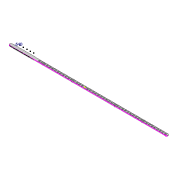
# Autodesk Inventor part: secondbow
Saved by Autodesk Inventor 2017 (Build 210142000, 142)
## iProperties
Created: 2017-04-15
Part Number: secondbow
Material: Generic
Document SubType Name: Modeling
Designer: Gideon
Density: 1 g/cm^3
Appearance: Default
Author: Gideon
Autodesk Inventor part; units mm, degrees
ref_plane "YZ Plane" through (0, 0, 0) normal (1, 0, 0) x (0, 1, 0)
ref_plane "XZ Plane" through (0, 0, 0) normal (0, 1, 0) x (-1, 0, 0)
ref_plane "XY Plane" through (0, 0, 0) normal (0, 0, 1) x (1, 0, 0)
sketch "Sketch1" plane through (0, 0, 0) normal (0, 0, 1) x (1, 0, 0)
  line L0 (-354.9792, 6.35) -> (394.3208, 6.35)
  line L1 (394.3208, 6.35) -> (394.3208, -6.35)
  line L2 (394.3208, -6.35) -> (-354.9792, -6.35)
  line L3 (-354.9792, -6.35) -> (-354.9792, 6.35)
  line L4 (-410.3367, 0) -> (469.0371, 0)
  point P0 (0, 0)
  dimension "d0" = 749.3
  dimension "d1" = 12.7
  constraints: 10 end point, 2 horizontal, 2 parallel, 1 perpendicular, 1 other
  measures "d0" distance of L0.end L0.start
  measures "d1" distance of L2.end L0.start
extrude "Extrusion1" add sketch "Sketch1" along normal blind 7.62
sketch "Sketch2" plane through (0, 0, 7.62) normal (0, 0, 1) x (1, 0, 0)
  line L0 (379.0808, 3.8322) -> (386.7008, 3.8322)
  line L1 (386.7008, 3.8322) -> (386.7008, -3.7878)
  line L2 (386.7008, -3.7878) -> (379.0808, -3.7878)
  line L3 (379.0808, -3.7878) -> (379.0808, 3.8322)
  line L4 (394.3208, -6.35) -> (394.3208, 6.35) projected
  line L5 (359.1521, 0.0222) -> (400.4054, 0.0222)
  line L6 (366.3808, -3.7878) -> (366.3808, 3.8322)
  line L7 (366.3808, 3.8322) -> (374.0008, 3.8322)
  line L8 (374.0008, 3.8322) -> (374.0008, -3.7878)
  line L9 (374.0008, -3.7878) -> (366.3808, -3.7878)
  line L10 (353.6808, -3.7878) -> (353.6808, 3.8322)
  line L11 (353.6808, 3.8322) -> (361.3008, 3.8322)
  line L12 (361.3008, 3.8322) -> (361.3008, -3.7878)
  line L13 (361.3008, -3.7878) -> (353.6808, -3.7878)
  line L14 (340.9808, -3.7878) -> (340.9808, 3.8322)
  line L15 (340.9808, 3.8322) -> (348.6008, 3.8322)
  line L16 (348.6008, 3.8322) -> (348.6008, -3.7878)
  line L17 (348.6008, -3.7878) -> (340.9808, -3.7878)
  line L18 (328.2808, -3.7878) -> (328.2808, 3.8322)
  line L19 (328.2808, 3.8322) -> (335.9008, 3.8322)
  line L20 (335.9008, 3.8322) -> (335.9008, -3.7878)
  line L21 (335.9008, -3.7878) -> (328.2808, -3.7878)
  line L22 (315.5808, -3.7878) -> (315.5808, 3.8322)
  line L23 (315.5808, 3.8322) -> (323.2008, 3.8322)
  line L24 (323.2008, 3.8322) -> (323.2008, -3.7878)
  line L25 (323.2008, -3.7878) -> (315.5808, -3.7878)
  line L26 (302.8808, -3.7878) -> (302.8808, 3.8322)
  line L27 (302.8808, 3.8322) -> (310.5008, 3.8322)
  line L28 (310.5008, 3.8322) -> (310.5008, -3.7878)
  line L29 (310.5008, -3.7878) -> (302.8808, -3.7878)
  line L30 (290.1808, -3.7878) -> (290.1808, 3.8322)
  line L31 (290.1808, 3.8322) -> (297.8008, 3.8322)
  line L32 (297.8008, 3.8322) -> (297.8008, -3.7878)
  line L33 (297.8008, -3.7878) -> (290.1808, -3.7878)
  line L34 (277.4808, -3.7878) -> (277.4808, 3.8322)
  line L35 (277.4808, 3.8322) -> (285.1008, 3.8322)
  line L36 (285.1008, 3.8322) -> (285.1008, -3.7878)
  line L37 (285.1008, -3.7878) -> (277.4808, -3.7878)
  line L38 (264.7808, -3.7878) -> (264.7808, 3.8322)
  line L39 (264.7808, 3.8322) -> (272.4008, 3.8322)
  line L40 (272.4008, 3.8322) -> (272.4008, -3.7878)
  line L41 (272.4008, -3.7878) -> (264.7808, -3.7878)
  line L42 (252.0808, -3.7878) -> (252.0808, 3.8322)
  line L43 (252.0808, 3.8322) -> (259.7008, 3.8322)
  line L44 (259.7008, 3.8322) -> (259.7008, -3.7878)
  line L45 (259.7008, -3.7878) -> (252.0808, -3.7878)
  line L46 (239.3808, -3.7878) -> (239.3808, 3.8322)
  line L47 (239.3808, 3.8322) -> (247.0008, 3.8322)
  line L48 (247.0008, 3.8322) -> (247.0008, -3.7878)
  line L49 (247.0008, -3.7878) -> (239.3808, -3.7878)
  line L50 (226.6808, -3.7878) -> (226.6808, 3.8322)
  line L51 (226.6808, 3.8322) -> (234.3008, 3.8322)
  line L52 (234.3008, 3.8322) -> (234.3008, -3.7878)
  line L53 (234.3008, -3.7878) -> (226.6808, -3.7878)
  line L54 (213.9808, -3.7878) -> (213.9808, 3.8322)
  line L55 (213.9808, 3.8322) -> (221.6008, 3.8322)
  line L56 (221.6008, 3.8322) -> (221.6008, -3.7878)
  line L57 (221.6008, -3.7878) -> (213.9808, -3.7878)
  line L58 (201.2808, -3.7878) -> (201.2808, 3.8322)
  line L59 (201.2808, 3.8322) -> (208.9008, 3.8322)
  line L60 (208.9008, 3.8322) -> (208.9008, -3.7878)
  line L61 (208.9008, -3.7878) -> (201.2808, -3.7878)
  line L62 (188.5808, -3.7878) -> (188.5808, 3.8322)
  line L63 (188.5808, 3.8322) -> (196.2008, 3.8322)
  line L64 (196.2008, 3.8322) -> (196.2008, -3.7878)
  line L65 (196.2008, -3.7878) -> (188.5808, -3.7878)
  line L66 (175.8808, -3.7878) -> (175.8808, 3.8322)
  line L67 (175.8808, 3.8322) -> (183.5008, 3.8322)
  line L68 (183.5008, 3.8322) -> (183.5008, -3.7878)
  line L69 (183.5008, -3.7878) -> (175.8808, -3.7878)
  line L70 (163.1808, -3.7878) -> (163.1808, 3.8322)
  line L71 (163.1808, 3.8322) -> (170.8008, 3.8322)
  line L72 (170.8008, 3.8322) -> (170.8008, -3.7878)
  line L73 (170.8008, -3.7878) -> (163.1808, -3.7878)
  line L74 (150.4808, -3.7878) -> (150.4808, 3.8322)
  line L75 (150.4808, 3.8322) -> (158.1008, 3.8322)
  line L76 (158.1008, 3.8322) -> (158.1008, -3.7878)
  line L77 (158.1008, -3.7878) -> (150.4808, -3.7878)
  line L78 (137.7808, -3.7878) -> (137.7808, 3.8322)
  line L79 (137.7808, 3.8322) -> (145.4008, 3.8322)
  line L80 (145.4008, 3.8322) -> (145.4008, -3.7878)
  line L81 (145.4008, -3.7878) -> (137.7808, -3.7878)
  line L82 (125.0808, -3.7878) -> (125.0808, 3.8322)
  line L83 (125.0808, 3.8322) -> (132.7008, 3.8322)
  line L84 (132.7008, 3.8322) -> (132.7008, -3.7878)
  line L85 (132.7008, -3.7878) -> (125.0808, -3.7878)
  line L86 (112.3808, -3.7878) -> (112.3808, 3.8322)
  line L87 (112.3808, 3.8322) -> (120.0008, 3.8322)
  line L88 (120.0008, 3.8322) -> (120.0008, -3.7878)
  line L89 (120.0008, -3.7878) -> (112.3808, -3.7878)
  line L90 (99.6808, -3.7878) -> (99.6808, 3.8322)
  line L91 (99.6808, 3.8322) -> (107.3008, 3.8322)
  line L92 (107.3008, 3.8322) -> (107.3008, -3.7878)
  line L93 (107.3008, -3.7878) -> (99.6808, -3.7878)
  line L94 (86.9808, -3.7878) -> (86.9808, 3.8322)
  line L95 (86.9808, 3.8322) -> (94.6008, 3.8322)
  line L96 (94.6008, 3.8322) -> (94.6008, -3.7878)
  line L97 (94.6008, -3.7878) -> (86.9808, -3.7878)
  line L98 (74.2808, -3.7878) -> (74.2808, 3.8322)
  line L99 (74.2808, 3.8322) -> (81.9008, 3.8322)
  line L100 (81.9008, 3.8322) -> (81.9008, -3.7878)
  line L101 (81.9008, -3.7878) -> (74.2808, -3.7878)
  line L102 (61.5808, -3.7878) -> (61.5808, 3.8322)
  line L103 (61.5808, 3.8322) -> (69.2008, 3.8322)
  line L104 (69.2008, 3.8322) -> (69.2008, -3.7878)
  line L105 (69.2008, -3.7878) -> (61.5808, -3.7878)
  line L106 (48.8808, -3.7878) -> (48.8808, 3.8322)
  line L107 (48.8808, 3.8322) -> (56.5008, 3.8322)
  line L108 (56.5008, 3.8322) -> (56.5008, -3.7878)
  line L109 (56.5008, -3.7878) -> (48.8808, -3.7878)
  line L110 (36.1808, -3.7878) -> (36.1808, 3.8322)
  line L111 (36.1808, 3.8322) -> (43.8008, 3.8322)
  line L112 (43.8008, 3.8322) -> (43.8008, -3.7878)
  line L113 (43.8008, -3.7878) -> (36.1808, -3.7878)
  line L114 (23.4808, -3.7878) -> (23.4808, 3.8322)
  line L115 (23.4808, 3.8322) -> (31.1008, 3.8322)
  line L116 (31.1008, 3.8322) -> (31.1008, -3.7878)
  line L117 (31.1008, -3.7878) -> (23.4808, -3.7878)
  line L118 (10.7808, -3.7878) -> (10.7808, 3.8322)
  line L119 (10.7808, 3.8322) -> (18.4008, 3.8322)
  line L120 (18.4008, 3.8322) -> (18.4008, -3.7878)
  line L121 (18.4008, -3.7878) -> (10.7808, -3.7878)
  line L122 (-1.9192, -3.7878) -> (-1.9192, 3.8322)
  line L123 (-1.9192, 3.8322) -> (5.7008, 3.8322)
  line L124 (5.7008, 3.8322) -> (5.7008, -3.7878)
  line L125 (5.7008, -3.7878) -> (-1.9192, -3.7878)
  line L126 (-14.6192, -3.7878) -> (-14.6192, 3.8322)
  line L127 (-14.6192, 3.8322) -> (-6.9992, 3.8322)
  line L128 (-6.9992, 3.8322) -> (-6.9992, -3.7878)
  line L129 (-6.9992, -3.7878) -> (-14.6192, -3.7878)
  line L130 (-27.3192, -3.7878) -> (-27.3192, 3.8322)
  line L131 (-27.3192, 3.8322) -> (-19.6992, 3.8322)
  line L132 (-19.6992, 3.8322) -> (-19.6992, -3.7878)
  line L133 (-19.6992, -3.7878) -> (-27.3192, -3.7878)
  line L134 (-40.0192, -3.7878) -> (-40.0192, 3.8322)
  line L135 (-40.0192, 3.8322) -> (-32.3992, 3.8322)
  line L136 (-32.3992, 3.8322) -> (-32.3992, -3.7878)
  line L137 (-32.3992, -3.7878) -> (-40.0192, -3.7878)
  line L138 (-52.7192, -3.7878) -> (-52.7192, 3.8322)
  line L139 (-52.7192, 3.8322) -> (-45.0992, 3.8322)
  line L140 (-45.0992, 3.8322) -> (-45.0992, -3.7878)
  line L141 (-45.0992, -3.7878) -> (-52.7192, -3.7878)
  line L142 (-65.4192, -3.7878) -> (-65.4192, 3.8322)
  line L143 (-65.4192, 3.8322) -> (-57.7992, 3.8322)
  line L144 (-57.7992, 3.8322) -> (-57.7992, -3.7878)
  line L145 (-57.7992, -3.7878) -> (-65.4192, -3.7878)
  line L146 (-78.1192, -3.7878) -> (-78.1192, 3.8322)
  line L147 (-78.1192, 3.8322) -> (-70.4992, 3.8322)
  line L148 (-70.4992, 3.8322) -> (-70.4992, -3.7878)
  line L149 (-70.4992, -3.7878) -> (-78.1192, -3.7878)
  line L150 (-90.8192, -3.7878) -> (-90.8192, 3.8322)
  line L151 (-90.8192, 3.8322) -> (-83.1992, 3.8322)
  line L152 (-83.1992, 3.8322) -> (-83.1992, -3.7878)
  line L153 (-83.1992, -3.7878) -> (-90.8192, -3.7878)
  line L154 (-103.5192, -3.7878) -> (-103.5192, 3.8322)
  line L155 (-103.5192, 3.8322) -> (-95.8992, 3.8322)
  line L156 (-95.8992, 3.8322) -> (-95.8992, -3.7878)
  line L157 (-95.8992, -3.7878) -> (-103.5192, -3.7878)
  line L158 (-116.2192, -3.7878) -> (-116.2192, 3.8322)
  line L159 (-116.2192, 3.8322) -> (-108.5992, 3.8322)
  line L160 (-108.5992, 3.8322) -> (-108.5992, -3.7878)
  line L161 (-108.5992, -3.7878) -> (-116.2192, -3.7878)
  line L162 (-128.9192, -3.7878) -> (-128.9192, 3.8322)
  line L163 (-128.9192, 3.8322) -> (-121.2992, 3.8322)
  line L164 (-121.2992, 3.8322) -> (-121.2992, -3.7878)
  line L165 (-121.2992, -3.7878) -> (-128.9192, -3.7878)
  line L166 (-141.6192, -3.7878) -> (-141.6192, 3.8322)
  line L167 (-141.6192, 3.8322) -> (-133.9992, 3.8322)
  line L168 (-133.9992, 3.8322) -> (-133.9992, -3.7878)
  line L169 (-133.9992, -3.7878) -> (-141.6192, -3.7878)
  line L170 (-154.3192, -3.7878) -> (-154.3192, 3.8322)
  line L171 (-154.3192, 3.8322) -> (-146.6992, 3.8322)
  line L172 (-146.6992, 3.8322) -> (-146.6992, -3.7878)
  line L173 (-146.6992, -3.7878) -> (-154.3192, -3.7878)
  line L174 (-167.0192, -3.7878) -> (-167.0192, 3.8322)
  line L175 (-167.0192, 3.8322) -> (-159.3992, 3.8322)
  line L176 (-159.3992, 3.8322) -> (-159.3992, -3.7878)
  line L177 (-159.3992, -3.7878) -> (-167.0192, -3.7878)
  line L178 (-179.7192, -3.7878) -> (-179.7192, 3.8322)
  line L179 (-179.7192, 3.8322) -> (-172.0992, 3.8322)
  line L180 (-172.0992, 3.8322) -> (-172.0992, -3.7878)
  line L181 (-172.0992, -3.7878) -> (-179.7192, -3.7878)
  line L182 (-192.4192, -3.7878) -> (-192.4192, 3.8322)
  line L183 (-192.4192, 3.8322) -> (-184.7992, 3.8322)
  line L184 (-184.7992, 3.8322) -> (-184.7992, -3.7878)
  line L185 (-184.7992, -3.7878) -> (-192.4192, -3.7878)
  line L186 (-205.1192, -3.7878) -> (-205.1192, 3.8322)
  line L187 (-205.1192, 3.8322) -> (-197.4992, 3.8322)
  line L188 (-197.4992, 3.8322) -> (-197.4992, -3.7878)
  line L189 (-197.4992, -3.7878) -> (-205.1192, -3.7878)
  line L190 (-217.8192, -3.7878) -> (-217.8192, 3.8322)
  line L191 (-217.8192, 3.8322) -> (-210.1992, 3.8322)
  line L192 (-210.1992, 3.8322) -> (-210.1992, -3.7878)
  line L193 (-210.1992, -3.7878) -> (-217.8192, -3.7878)
  point P0 (0, 0)
  dimension "d6" = 7.62
  dimension "d7" = 7.62
  dimension "d8" = 7.62
  dimension "d11" = 12.7
  constraints: 386 end point, 2 horizontal, 2 parallel, 2 perpendicular, 377 other
  measures "d6" distance of L0.end L0.start
  measures "d7" distance of L1.end L0.end
  measures "d8" distance from line of L4 L0.end
  measures "d11" distance of L2.end L6.start
extrude "Extrusion2" cut sketch "Sketch2" against normal blind 3.81
sketch "Sketch3" plane through (0, 0, 7.62) normal (0, 0, 1) x (1, 0, 0)
  point P0 (0, 0)
sketch "Sketch4" plane through (0, 0, 7.62) normal (0, 0, 1) x (1, 0, 0)
  line L0 (-348.6292, -6.35) -> (394.3208, -6.35) projected
  arc A0 (-348.6292, -6.35) -> (-333.0842, -6.35) centre (-340.8567, 18.9748) ccw
  arc A1 (-332.3732, -6.35) -> (-316.8282, -6.35) centre (-324.6007, 18.9748) ccw
  arc A2 (-316.1172, -6.35) -> (-300.5722, -6.35) centre (-308.3447, 18.9748) ccw
  arc A3 (-299.8612, -6.35) -> (-284.3162, -6.35) centre (-292.0887, 18.9748) ccw
  arc A4 (-283.6052, -6.35) -> (-268.0602, -6.35) centre (-275.8327, 18.9748) ccw
  arc A5 (-267.3492, -6.35) -> (-251.8042, -6.35) centre (-259.5767, 18.9748) ccw
  point P0 (0, 0)
  point P1 (387.9708, -6.35)
  dimension "d23" = 16.256
  constraints: 12 point on circle, 6 centre point, 1 horizontal, 1 point on line, 20 other
  measures "d23" distance of A0.centre A1.centre
sketch "Sketch5" plane through (0, 0, 7.62) normal (0, 0, 1) x (1, 0, 0)
  arc A0 (-348.6292, -6.35) -> (-332.6522, -6.35) centre (-340.6407, 18.9075) ccw projected
  line L0 (-348.6292, -6.35) -> (394.3208, -6.35) projected
  line L1 (-332.6522, -6.35) -> (-332.6522, 6.35) projected
  arc A1 (-332.6522, -6.35) -> (-316.6552, -6.35) centre (-324.6537, 18.4514) ccw
  point P0 (0, 0)
  point P1 (387.9708, -6.35)
  dimension "d30" = 15.997
  constraints: 2 point on circle, 1 centre point, 1 point on line
  measures "d30" distance of L1.start A1.end
sketch "Sketch6" plane through (0, 0, 7.62) normal (0, 0, 1) x (1, 0, 0)
  arc A0 (-332.6522, -6.35) -> (-316.6552, -6.35) centre (-324.6537, 18.4514) ccw projected
  line L0 (-348.6292, -6.35) -> (394.3208, -6.35) projected
  arc A1 (-316.6552, -6.35) -> (-300.6582, -6.35) centre (-308.6567, 18.4264) ccw
  point P0 (0, 0)
  point P1 (387.9708, -6.35)
  dimension "d33" = 15.997
  constraints: 2 point on circle, 1 centre point, 1 point on line
  measures "d33" distance of A0.end A1.end
sketch "Sketch7" plane through (0, 0, 7.62) normal (0, 0, 1) x (1, 0, 0)
  arc A0 (-316.6552, -6.35) -> (-300.6582, -6.35) centre (-308.6567, 18.4264) ccw projected
  line L0 (-348.6292, -6.35) -> (394.3208, -6.35) projected
  arc A1 (-300.6582, -6.35) -> (-284.6612, -6.35) centre (-292.6597, 18.3368) ccw
  point P0 (0, 0)
  point P1 (387.9708, -6.35)
  dimension "d36" = 15.997
  constraints: 2 point on circle, 1 centre point, 1 point on line
  measures "d36" distance of A0.end A1.end
sketch "Sketch8" plane through (0, 0, 7.62) normal (0, 0, 1) x (1, 0, 0)
  arc A0 (-300.6582, -6.35) -> (-284.6612, -6.35) centre (-292.6597, 18.3368) ccw projected
  line L0 (-348.6292, -6.35) -> (394.3208, -6.35) projected
  arc A1 (-284.6612, -6.35) -> (-268.6642, -6.35) centre (-276.6627, 18.2987) ccw
  point P0 (0, 0)
  point P1 (387.9708, -6.35)
  dimension "d39" = 15.997
  constraints: 2 point on circle, 1 centre point, 1 point on line
  measures "d39" distance of A0.end A1.end
sketch "Sketch9" plane through (0, 0, 7.62) normal (0, 0, 1) x (1, 0, 0)
  arc A0 (-284.6612, -6.35) -> (-268.6642, -6.35) centre (-276.6627, 18.2987) ccw projected
  line L0 (-348.6292, -6.35) -> (394.3208, -6.35) projected
  arc A1 (-268.6642, -6.35) -> (-252.6672, -6.35) centre (-260.6657, 18.2707) ccw
  point P0 (0, 0)
  point P1 (387.9708, -6.35)
  dimension "d42" = 15.997
  constraints: 2 point on circle, 1 centre point, 1 point on line
  measures "d42" distance of A0.end A1.end
sketch "Sketch10" plane through (0, 0, 7.62) normal (0, 0, 1) x (1, 0, 0)
  arc A0 (-268.6642, -6.35) -> (-252.6672, -6.35) centre (-260.6657, 18.2707) ccw projected
  line L0 (-252.6672, -6.35) -> (-252.6672, 6.35) projected
  line L1 (-348.6292, -6.35) -> (394.3208, -6.35) projected
  arc A1 (-252.6672, -6.35) -> (-236.6702, -6.35) centre (-244.6687, 17.8049) ccw
  point P0 (0, 0)
  point P1 (387.9708, -6.35)
  dimension "d45" = 15.997
  constraints: 2 point on circle, 1 centre point, 1 point on line
  measures "d45" distance of L0.start A1.end
fillet "Fillet4" radius 6.35 2 edges at (19.6708, 6.35, 0) (19.6708, -6.35, 0)
fillet "Fillet5" radius 6.35 3 edges at (394.3208, -6.35, 6.9849) (394.3208, 6.35, 6.9849) (394.3208, 4.4902, 1.8598)
fillet "Fillet6" radius 6.35 3 edges at (-354.9792, 4.4902, 1.8598) (-354.9792, 6.35, 6.9849) (-354.9792, -6.35, 6.9849)
sketch "Sketch17" plane through (0, 0, 7.62) normal (0, 0, 1) x (1, 0, 0)
  point P0 (0, 0)
sketch3d "3D Sketch8"
  line L0 (-348.6292, -6.35, 7.62) -> (-348.6292, -6.35, 6.35)
  arc A0 (-348.6292, 6.35, 6.35) -> (-348.6292, 4.4901, 1.8599) centre (-348.6292, 0, 6.35) ccw
  arc A1 (-348.6292, 4.4901, 1.8599) -> (-348.6292, 0, 0) centre (-348.6292, 0, 6.35) ccw
  arc A2 (-348.6292, 0, 0) -> (-348.6292, -4.4901, 1.8599) centre (-348.6292, 0, 6.35) ccw
  arc A3 (-348.6292, -4.4901, 1.8599) -> (-348.6292, -6.35, 6.35) centre (-348.6292, 0, 6.35) ccw
  line L1 (-348.6292, 6.35, 6.35) -> (-348.6292, 6.35, 7.62)
  constraints: 3 horizontal
sweep "Sweep8" add profiles "Sketch5" path "3D Sketch8" contours L0 A0
sketch3d "3D Sketch9"
  line L0 (-348.6292, -6.35, 7.62) -> (-348.6292, -6.35, 6.35)
  arc A0 (-348.6292, 6.35, 6.35) -> (-348.6292, 4.4901, 1.8599) centre (-348.6292, 0, 6.35) ccw
  arc A1 (-348.6292, 4.4901, 1.8599) -> (-348.6292, 0, 0) centre (-348.6292, 0, 6.35) ccw
  arc A2 (-348.6292, 0, 0) -> (-348.6292, -4.4901, 1.8599) centre (-348.6292, 0, 6.35) ccw
  arc A3 (-348.6292, -4.4901, 1.8599) -> (-348.6292, -6.35, 6.35) centre (-348.6292, 0, 6.35) ccw
  line L1 (-348.6292, 6.35, 6.35) -> (-348.6292, 6.35, 7.62)
  constraints: 3 horizontal
sweep "Sweep9" add profiles "Sketch6" path "3D Sketch9" contours L0 A1
sketch3d "3D Sketch10"
  line L0 (-348.6292, -6.35, 7.62) -> (-348.6292, -6.35, 6.35)
  arc A0 (-348.6292, 6.35, 6.35) -> (-348.6292, 4.4901, 1.8599) centre (-348.6292, 0, 6.35) ccw
  arc A1 (-348.6292, 4.4901, 1.8599) -> (-348.6292, 0, 0) centre (-348.6292, 0, 6.35) ccw
  arc A2 (-348.6292, 0, 0) -> (-348.6292, -4.4901, 1.8599) centre (-348.6292, 0, 6.35) ccw
  arc A3 (-348.6292, -4.4901, 1.8599) -> (-348.6292, -6.35, 6.35) centre (-348.6292, 0, 6.35) ccw
  line L1 (-348.6292, 6.35, 6.35) -> (-348.6292, 6.35, 7.62)
  constraints: 3 horizontal
sweep "Sweep10" add profiles "Sketch7" path "3D Sketch10" contours L0 A1
sketch3d "3D Sketch11"
  line L0 (-348.6292, -6.35, 7.62) -> (-348.6292, -6.35, 6.35)
  arc A0 (-348.6292, 6.35, 6.35) -> (-348.6292, 4.4901, 1.8599) centre (-348.6292, 0, 6.35) ccw
  arc A1 (-348.6292, 4.4901, 1.8599) -> (-348.6292, 0, 0) centre (-348.6292, 0, 6.35) ccw
  arc A2 (-348.6292, 0, 0) -> (-348.6292, -4.4901, 1.8599) centre (-348.6292, 0, 6.35) ccw
  arc A3 (-348.6292, -4.4901, 1.8599) -> (-348.6292, -6.35, 6.35) centre (-348.6292, 0, 6.35) ccw
  line L1 (-348.6292, 6.35, 6.35) -> (-348.6292, 6.35, 7.62)
  constraints: 3 horizontal
sweep "Sweep11" add profiles "Sketch8" path "3D Sketch11" contours L0 A1
sketch3d "3D Sketch12"
  line L0 (-348.6292, -6.35, 7.62) -> (-348.6292, -6.35, 6.35)
  arc A0 (-348.6292, 6.35, 6.35) -> (-348.6292, 4.4901, 1.8599) centre (-348.6292, 0, 6.35) ccw
  arc A1 (-348.6292, 4.4901, 1.8599) -> (-348.6292, 0, 0) centre (-348.6292, 0, 6.35) ccw
  arc A2 (-348.6292, 0, 0) -> (-348.6292, -4.4901, 1.8599) centre (-348.6292, 0, 6.35) ccw
  arc A3 (-348.6292, -4.4901, 1.8599) -> (-348.6292, -6.35, 6.35) centre (-348.6292, 0, 6.35) ccw
  line L1 (-348.6292, 6.35, 6.35) -> (-348.6292, 6.35, 7.62)
  constraints: 3 horizontal
sweep "Sweep12" add profiles "Sketch9" path "3D Sketch12" contours L0 A1
sketch3d "3D Sketch13"
  line L0 (-348.6292, -6.35, 7.62) -> (-348.6292, -6.35, 6.35)
  arc A0 (-348.6292, 6.35, 6.35) -> (-348.6292, 4.4901, 1.8599) centre (-348.6292, 0, 6.35) ccw
  arc A1 (-348.6292, 4.4901, 1.8599) -> (-348.6292, 0, 0) centre (-348.6292, 0, 6.35) ccw
  arc A2 (-348.6292, 0, 0) -> (-348.6292, -4.4901, 1.8599) centre (-348.6292, 0, 6.35) ccw
  arc A3 (-348.6292, -4.4901, 1.8599) -> (-348.6292, -6.35, 6.35) centre (-348.6292, 0, 6.35) ccw
  line L1 (-348.6292, 6.35, 6.35) -> (-348.6292, 6.35, 7.62)
  constraints: 3 horizontal
sweep "Sweep13" add profiles "Sketch10" path "3D Sketch13" contours L1 A1
sketch "Sketch18" plane through (0, 0, 7.62) normal (0, 0, 1) x (1, 0, 0)
  line L0 (-332.6522, -6.35) -> (-316.6552, -6.35) projected
  arc A0 (-316.6552, -6.35) -> (-300.6582, -6.35) centre (-308.6567, 18.4264) ccw projected
  arc A1 (-332.6522, -6.35) -> (-316.6552, -6.35) centre (-324.6537, 15.2524) ccw
  point P0 (0, 0)
  constraints: 2 point on circle, 1 centre point
sketch3d "3D Sketch14"
  line L0 (-348.6292, -6.35, 7.62) -> (-348.6292, -6.35, 6.35)
  arc A0 (-348.6292, 6.35, 6.35) -> (-348.6292, 4.4901, 1.8599) centre (-348.6292, 0, 6.35) ccw
  arc A1 (-348.6292, 4.4901, 1.8599) -> (-348.6292, 0, 0) centre (-348.6292, 0, 6.35) ccw
  arc A2 (-348.6292, 0, 0) -> (-348.6292, -4.4901, 1.8599) centre (-348.6292, 0, 6.35) ccw
  arc A3 (-348.6292, -4.4901, 1.8599) -> (-348.6292, -6.35, 6.35) centre (-348.6292, 0, 6.35) ccw
  line L1 (-348.6292, 6.35, 6.35) -> (-348.6292, 6.35, 7.62)
  constraints: 3 horizontal
sweep "Sweep14" add profiles "Sketch18" path "3D Sketch14"
sketch "Sketch23" plane through (0, 0, 7.62) normal (0, 0, 1) x (1, 0, 0)
  line L0 (-194.7142, 9.3835) -> (-194.7142, -15.5443)
  point P0 (0, 0)
  constraints: 2 end point, 1 vertical
split body "Split10" sketch "Sketch23" result two bodies curves L0 first body at (193.7425, -4.8335, 3.0545)
sketch "Sketch24" plane through (0, 0, 7.62) normal (0, 0, 1) x (1, 0, 0)
  line L0 (-55.4474, 12.5465) -> (-55.4474, -13.7607)
  point P0 (0, 0)
  constraints: 2 end point, 1 vertical
split body "Split11" sketch "Sketch24" result two bodies bodies 2 curves L0 first body at (92.3587, 5.7847, 5.478)
sketch "Sketch25" plane through (0, 0, 7.62) normal (0, 0, 1) x (1, 0, 0)
  line L0 (146.7822, 9.2091) -> (146.7822, -19.7683)
  point P0 (0, 0)
  constraints: 2 end point, 1 vertical
split body "Split12" sketch "Sketch25" result two bodies bodies 4 curves L0 first body at (307.5746, -5.0663, 3.4249)
sketch "Sketch26" plane through (0, 0, 7.62) normal (0, 0, 1) x (1, 0, 0)
  line L0 (274.5771, 8.7169) -> (274.5771, -13.5304)
  line L1 (146.7822, 6.35) -> (387.9708, 6.35) projected
  point P0 (0, 0)
  constraints: 2 end point, 1 perpendicular
split body "Split13" sketch "Sketch26" result two bodies bodies 6 curves L0 first body at (350.173, -5.0663, 3.4249)
body "Solid19"
body "Solid21"
body "Solid23"
body "Solid24"
body "Solid25"
